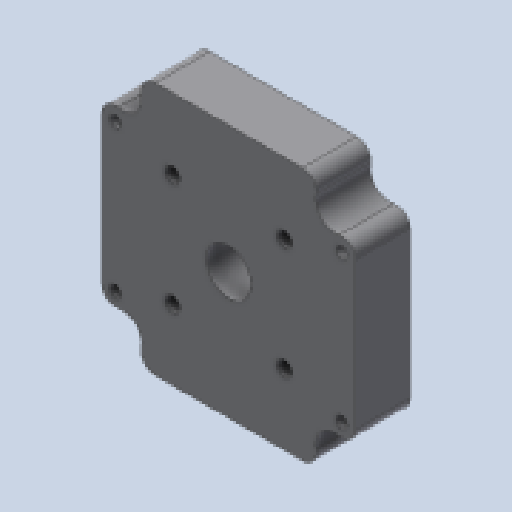
# Autodesk Inventor part: NeckEncoderMount
Saved by Autodesk Inventor 2025.2 (Build 292293000, 293)
## iProperties
Created: 2026-01-18
Part Number: NeckEncoderMount
Material: Generic
Document SubType Name: Sheet Metal
Designer: valer
Density: 1 g/cm^3
Sheet Metal Rule: Default
Appearance: Default
Author: valer
Autodesk Inventor part; units mm, degrees
ref_plane "YZ Plane" through (0, 0, 0) normal (1, 0, 0) x (0, 1, 0)
ref_plane "XZ Plane" through (0, 0, 0) normal (0, 1, 0) x (-1, 0, 0)
ref_plane "XY Plane" through (0, 0, 0) normal (0, 0, 1) x (1, 0, 0)
sketch "Base" plane through (0, 0, 0) normal (0, 0, 1) x (1, 0, 0)
  circle A0 centre (18.3354, -21.8597) radius 1.2295
  circle A1 centre (-31.6646, -21.8597) radius 1.2295
  circle A2 centre (18.3354, 10.6981) radius 1.2295
  circle A3 centre (-31.6646, 10.6981) radius 1.2295
  circle A4 centre (-6.6646, -5.5808) radius 5
  arc A5 (21.3354, 10.6981) -> (17.758, 13.642) centre (18.3354, 10.6981) ccw
  arc A6 (12.5583, 18.8418) -> (17.758, 13.642) centre (16.9054, 17.9892) ccw
  arc A7 (12.5583, 18.8418) -> (9.6143, 22.4192) centre (9.6143, 19.4192) ccw
  line L0 (9.6143, 22.4192) -> (-22.9435, 22.4192)
  arc A8 (-22.9435, 22.4192) -> (-25.8874, 18.8418) centre (-22.9435, 19.4192) ccw
  arc A9 (-31.0872, 13.642) -> (-25.8874, 18.8418) centre (-30.2346, 17.9892) ccw
  arc A10 (-31.0872, 13.642) -> (-34.6646, 10.6981) centre (-31.6646, 10.6981) ccw
  line L1 (-34.6646, 10.6981) -> (-34.6646, -21.8597)
  arc A11 (-34.6646, -21.8597) -> (-31.0872, -24.8036) centre (-31.6646, -21.8597) ccw
  arc A12 (-25.8874, -30.0034) -> (-31.0872, -24.8036) centre (-30.2346, -29.1508) ccw
  arc A13 (-25.8874, -30.0034) -> (-22.9435, -33.5808) centre (-22.9435, -30.5808) ccw
  line L2 (-22.9435, -33.5808) -> (9.6143, -33.5808)
  arc A14 (9.6143, -33.5808) -> (12.5583, -30.0034) centre (9.6143, -30.5808) ccw
  arc A15 (17.758, -24.8036) -> (12.5583, -30.0034) centre (16.9054, -29.1508) ccw
  arc A16 (17.758, -24.8036) -> (21.3354, -21.8597) centre (18.3354, -21.8597) ccw
  line L3 (21.3354, -21.8597) -> (21.3354, 10.6981)
  circle A17 centre (-19.0581, -17.9611) radius 1.6234
  circle A18 centre (-19.0582, 6.7882) radius 1.6241
  circle A19 centre (5.6908, 6.7877) radius 1.6234
  circle A20 centre (5.6907, -17.9611) radius 1.6235
  point P0 (0, 0)
extrude "Plate1" add sketch "Base" along normal blind 12
equation "\"d0\" = Thickness"
equation "\"BendRadius\" = Thickness"
equation "\"BendReliefWidth\" = Thickness"
equation "\"BendReliefDepth\" = 0.5 * Thickness"
equation "\"CornerReliefSize\" = 4 * Thickness"
equation "\"MinimumRemnant\" = 2 * Thickness"
equation "\"TransitionRadius\" = BendRadius"
equation "\"JacobiRadiusSize\" = BendRadius"
equation "\"GapSize\" = Thickness"
equation "\"Thickness\" = 12"
body "Solid1"
